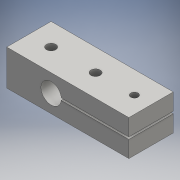
# Autodesk Inventor part: Lezerlefogov3
Saved by Autodesk Inventor 2016 (Build 200138000, 138)
## iProperties
Created: 2018-03-22
Part Number: Lezerlefogov3
Material: Generic
Document SubType Name: Modeling
Designer: bogna
Density: 1 g/cm^3
Appearance: Default
Author: bogna
Autodesk Inventor part; units mm, degrees
ref_plane "YZ Plane" through (0, 0, 0) normal (1, 0, 0) x (0, 1, 0)
ref_plane "XZ Plane" through (0, 0, 0) normal (0, 1, 0) x (-1, 0, 0)
sketch "Sketch1" plane through (0, 0, 0) normal (0, 0, 1) x (1, 0, 0)
  line L0 (-20, 10) -> (35, 10)
  line L1 (35, 10) -> (35, -10)
  line L2 (35, -10) -> (-20, -10)
  line L3 (-20, -10) -> (-20, 10)
  line L4 (-31, 0) -> (46, 0) projected
  line L5 (0, -14) -> (0, 14) projected
  point P0 (0, 0)
  point P1 (-10, 0)
  point P2 (10, 0)
  point P3 (27.5, 0)
  dimension "d0" = 20
  dimension "d2" = 55
  dimension "d8" = 20
  dimension "d9" = 20
  dimension "d10" = 7.5
  constraints: 8 end point, 3 point on line, 2 parallel, 1 horizontal, 1 perpendicular, 1 symmetric about line, 1 other
  measures "d0" distance of L2.end L0.start
  measures "d2" distance between parallel lines of L1 L3
  measures "d8" distance between parallel lines of L3 L5
  measures "d9" distance of point (10, 0) point (-10, 0)
  measures "d10" distance from line of L1 point (27.5, 0)
extrude "Extrusion1" add sketch "Sketch1" along normal blind 16
sketch "Sketch2" plane through (0, 0, 0) normal (0, 0, 1) x (1, 0, 0)
  line L0 (-20, 10) -> (35, 10)
  line L1 (35, 10) -> (35, -10)
  line L2 (35, -10) -> (-20, -10)
  line L3 (-20, -10) -> (-20, 10)
  line L4 (0, 14) -> (0, -14) projected
  line L5 (-31, 0) -> (46, 0) projected
  point P0 (0, 0)
  point P1 (-10, 0)
  point P2 (10, 0)
  dimension "d38" = 20
  dimension "d39" = 55
  dimension "d41" = 20
  constraints: 8 end point, 2 parallel, 1 horizontal, 1 perpendicular
  measures "d38" distance of L2.end L0.start
  measures "d39" distance between parallel lines of L1 L3
  measures "d41" distance of point (10, 0) point (-10, 0)
hole "Hole4" at (-10, 0, 0) at (10, 0, 0) direction (0, 0, 1) diameter 4.2 end through all counterbore diameter 8.65 counterbore depth 12.8
sketch "Sketch3" plane through (0, 0, 0) normal (0, 0, 1) x (1, 0, 0)
  line L0 (-20, 10) -> (35, 10)
  line L1 (35, 10) -> (35, -10)
  line L2 (35, -10) -> (-20, -10)
  line L3 (-20, -10) -> (-20, 10)
  point P0 (0, 0)
  point P1 (-10, 0)
  point P2 (10, 0)
  point P3 (27.5, 0)
  dimension "d50" = 20
  dimension "d51" = 55
  dimension "d52" = 20
  dimension "d53" = 7.5
  constraints: 8 end point, 2 parallel, 1 horizontal, 1 perpendicular
  measures "d50" distance of L2.end L0.start
  measures "d51" distance between parallel lines of L1 L3
  measures "d52" distance of point (10, 0) point (-10, 0)
  measures "d53" distance from line of L1 point (27.5, 0)
hole "Hole5" at (27.5, 0, 0) direction (0, 0, 1) diameter 4.2 depth 8 tip angle 118 counterbore diameter 8.65 counterbore depth 3.2
ref_plane "Work Plane1" through (0, 0, 8) normal (0, 0, -1) x (-1, 0, 0)
sketch "Sketch5" plane through (0, 0, 8) normal (0, 0, -1) x (-1, 0, 0)
  line L0 (-40, -10) -> (0, -10)
  line L1 (0, -10) -> (0, 10)
  line L2 (0, 10) -> (-40, 10)
  line L3 (-40, 10) -> (-40, -10)
  line L4 (49, 0) -> (-49, 0) projected
  line L5 (0, -14) -> (0, 14) projected
  point P0 (0, 0)
  point P1 (0, 0)
  dimension "d64" = 20
  dimension "d65" = 40
  constraints: 8 end point, 2 midpoint, 2 parallel, 1 horizontal, 1 perpendicular, 1 other
  measures "d64" distance of L0.end L1.end
  measures "d65" distance of L0.start L0.end
extrude "Extrusion2" cut sketch "Sketch5" along normal mid plane 1
sketch "Sketch6" plane through (0, 0, 0) normal (0, 1, 0) x (-1, 0, 0)
  line L0 (0, 7.5) -> (0, 8.5) projected
  circle A0 centre (0, 8) radius 4.6
  point P0 (0, 0)
  dimension "d68" = 9.2
  constraints: 1 centre point, 1 midpoint
  measures "d68" diameter of A0
extrude "Extrusion3" cut sketch "Sketch6" along normal mid plane 20
hole "Hole6" at (27.5, 0, 0) direction (0, 0, 1) diameter 3.3 end through all
body "Solid1"
